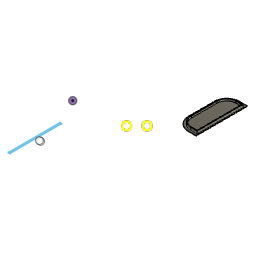
Enclosure2 (Autodesk Fusion 360 design; units mm, degrees)
Autodesk Fusion 360 part; units mm, degrees
sketch "Sketch1" plane through (0, 0, 0) normal (0, 0, 1) x (1, 0, 0) in component "Component"
sketch "Sketch2" plane through (0, 0, 0) normal (0, 0, 1) x (1, 0, 0) in component "Component"
  line L0 (75, -200) -> (70, -200)
  line L1 (50, -300) -> (55, -300)
  line L2 (55, -300) -> (55, -100)
  line L3 (55, -100) -> (50, -100)
  line L4 (50, -100) -> (50, -300)
  dimension "d13" = 5
  dimension "d14" = 200
  constraint horizontal L0
  constraint horizontal L1
  constraint vertical L2
  constraint horizontal L3
  constraint vertical L4
  measures "d13" distance of L1.start L1.end
  measures "d14" distance of L1.start L3.end
sketch "Sketch1 (2)" plane through (0, 0, 10) normal (0, 0, 1) x (-1, 0, 0) in component "Component'"
  arc A0 (-200, -10) -> (-240, -50) centre (-200, -50) ccw
sketch "Sketch1 (3)" plane through (0, 0, 0) normal (0, 0, 1) x (1, 0, 0) in component "Component''"
sketch "Sketch2 (2)" plane through (-95, 0, 0) normal (1, 0, 0) x (0, 1, 0) in component "Component''"
sketch "Sketch3" plane through (-100, 0, 0) normal (-1, 0, 0) x (0, -1, 0) in component "Component''"
sketch "Sketch4" plane through (0, 20, 0) normal (0, -1, 0) x (1, 0, 0) in component "Component''"
sketch "Sketch5" plane through (-20, 0, 0) normal (1, 0, 0) x (0, 1, 0) in component "Component''"
sketch "Sketch6" plane through (0, 20, 0) normal (0, -1, 0) x (1, 0, 0) in component "Component''"
sketch "Sketch7" plane through (0, 0, 0) normal (0, 0, 1) x (1, 0, 0) in component "Component''"
sketch "Sketch1 (4)" plane through (0, 0, 0) normal (0, 0, 1) x (1, 0, 0) in component "Component'''"
  line L0 (279.9422, 41.1483) -> (359.9422, 41.1483)
  line L1 (359.9422, 41.1483) -> (359.9422, 241.1483)
  line L2 (359.9422, 241.1483) -> (279.9422, 241.1483)
  line L3 (279.9422, 241.1483) -> (279.9422, 41.1483)
  dimension "d77" = 80
  dimension "d78" = 200
  constraint horizontal L0
  constraint vertical L1
  constraint horizontal L2
  constraint vertical L3
  measures "d77" distance of L0.start L0.end
  measures "d78" distance of L0.start L2.end
extrude "Extrude1" add sketch "Sketch1 (4)" along normal blind 2 makes body 1 in component "Component'''"
fillet "Fillet1" radius 50 1 edges at (279.9422, 41.1483, 1) on bodies 1 in component "Component'''"
fillet "Fillet2" radius 50 1 edges at (279.9422, 241.1483, 1) on bodies 1 in component "Component'''"
sketch "Sketch2 (3)" plane through (-100, 20, -90) normal (0, 0, 1) x (1, 0, 0) in component "Component'''"
  line L0 (75, 10) -> (10, 10)
  line L1 (10, 10) -> (10, 190)
  line L2 (10, 190) -> (75, 190)
  line L3 (75, 190) -> (75, 10)
  constraint horizontal L0
  constraint vertical L1
  constraint horizontal L2
  constraint vertical L3
extrude "Extrude2" add sketch "Sketch2 (3)" along normal blind 10 separate body makes body 2 in component "Component'''"
fillet "Fillet3" radius 40 1 edges at (-90, 30, -85) on bodies 2 in component "Component'''"
fillet "Fillet4" radius 40 1 edges at (-90, 210, -85) on bodies 2 in component "Component'''"
move_body "Move1" bodies 2 to x (1, 0, 0) y (0, 1, 0) z (0, 0, 1) at (380, 20, 90) in component "Component'''"
shell "Shell1" thickness 3 removed faces 1 at (333.3333, 123.3333, 10) on bodies 2 in component "Component'''"
component "Component" placed x (1, 0, 0) y (0, 1, 0) z (0, 0, 1) at (0.1052, -0.1574, 0)
component "Component'" placed x (1, 0, 0) y (0, 1, 0) z (0, 0, 1) at (0, 0, 0) in component "Component"
component "Component''" placed x (1, 0, 0) y (0, 1, 0) z (0, 0, 1) at (100, -20, 100) in component "Component'"
component "Component'''" placed x (1, 0, 0) y (0, 1, 0) z (0, 0, 1) at (0, 0, 0) in component "Component''"
